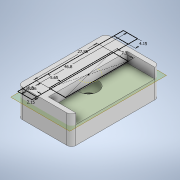
# Autodesk Inventor part: Capping_Parallelizer
Saved by Autodesk Inventor 2022 (Build 260153000, 153)
## iProperties
Created: 2024-04-15
Part Number: Capping_Parallelizer
Material: Generic
Document SubType Name: Modeling
Designer: Gotham City
Density: 1 g/cm^3
Appearance: Default
Author: Gotham City
Autodesk Inventor part; units mm, degrees
ref_plane "YZ Plane" through (0, 0, 0) normal (1, 0, 0) x (0, 1, 0)
ref_plane "XZ Plane" through (0, 0, 0) normal (0, 1, 0) x (-1, 0, 0)
sketch "Sketch1" plane through (0, 0, 0) normal (0, 1, 0) x (-1, 0, 0)
  line L0 (0, 0) -> (23.8, 0)
  line L1 (23.8, 0) -> (23.8, -39)
  line L2 (23.8, -39) -> (0, -39)
  line L3 (0, -39) -> (0, 0)
  circle A0 centre (11.9, -19.5) radius 9.9
  line L4 (23.8, 0) -> (0, -39) construction
  dimension "d0" = 19.8
  dimension "d1" = 11.9
  dimension "d2" = 39
  constraints: 10 end point, 2 parallel, 1 centre point, 1 coincident, 1 horizontal, 1 midpoint, 1 perpendicular
  measures "d0" diameter of A0
  measures "d1" distance from line of L1 A0.centre
  measures "d2" distance of L0.end L1.end
extrude "Extrusion1" add sketch "Sketch1" along normal blind 1.5
sketch "Sketch2" plane through (0, 0, 0) normal (0, -1, 0) x (1, 0, 0)
  line L0 (0, -39) -> (-23.8, -39) projected
  line L1 (0, 0) -> (0, -39) projected
  line L2 (-23.8, 0) -> (0, 0) projected
  line L3 (-23.8, -39) -> (-23.8, 0) projected
  circle A0 centre (-11.9, -19.5) radius 9.9 construction
  circle A1 centre (-11.9, -19.5) radius 4.25
  dimension "d5" = 8.5
  constraints: 1 centre point, 1 coincident
  measures "d5" diameter of A1
extrude "Extrusion2" add sketch "Sketch2" along normal blind 1
ref_plane "Work Plane1" through (0, 7, 0) normal (0, -1, 0) x (1, 0, 0)
sketch "Sketch4" plane through (0, 1.5, 0) normal (0, 1, 0) x (1, 0, 0)
  line L0 (0, 39) -> (-23.8, 39) projected
  line L1 (-23.8, 39) -> (-23.8, 0) projected
  line L2 (-23.8, 0) -> (0, 0) projected
  line L3 (0, 0) -> (0, 39) projected
  circle A0 centre (-11.9, 19.5) radius 4.25 projected
extrude "Extrusion3" add sketch "Sketch4" along normal up to surface (5.5 mm away)
sketch "Sketch5" plane through (-23.8, 7, -39) normal (0, 1, 0) x (1, 0, 0)
  line L0 (11.5916, -37) -> (27.5916, -37)
  line L1 (27.5916, -37) -> (27.5916, -2)
  line L2 (27.5916, -2) -> (11.5916, -2)
  line L3 (11.5916, -2) -> (11.5916, -37)
  line L4 (11.5916, -37) -> (27.5916, -2) construction
  line L5 (27.5916, -37) -> (11.5916, -2) construction
  line L6 (0, 0) -> (0, -39) projected
  line L7 (0, -39) -> (23.8, -39) projected
  line L8 (23.8, 0) -> (0, 0) projected
  line L9 (23.8, -39) -> (23.8, 0) projected
  dimension "d11" = 35
  dimension "d12" = 16
  constraints: 12 end point, 2 parallel, 1 horizontal, 1 perpendicular
  measures "d11" distance of L2.end L0.start
  measures "d12" distance of L0.start L0.end
extrude "Extrusion4" add sketch "Sketch5" along normal blind 4.5 contours L0 L9 L7 L6 L8 L2 L3
sketch "Sketch13" plane through (-23.8, 11.5, -39) normal (0, 1, 0) x (1, 0, 0)
  line L0 (8.9, -41.661) -> (2.6, -41.661)
  line L1 (2.6, -41.661) -> (2.6, 5.139)
  line L2 (2.6, 5.139) -> (8.9, 5.139)
  line L3 (8.9, 5.139) -> (8.9, -41.661)
  line L4 (8.25, -33.425) -> (8.25, -5.575) construction
  line L5 (15.55, -5.575) -> (8.25, -5.575)
  line L6 (8.25, -5.575) -> (8.25, -33.425)
  line L7 (8.25, -33.425) -> (15.55, -33.425)
  line L8 (15.55, -33.425) -> (15.55, -5.575)
  line L9 (15.55, -5.575) -> (8.25, -33.425) construction
  line L10 (8.25, -5.575) -> (15.55, -33.425) construction
  arc A0 (11.5916, -23.7388) -> (11.5916, -15.2612) centre (11.9, -19.5) ccw construction
  line L11 (2.6, 0.989) -> (8.9, 0.989)
  line L12 (8.9, -39.511) -> (2.6, -39.511)
  point P0 (11.9, -19.5)
  dimension "d62" = 5.65
  dimension "d63" = 46.8
  dimension "d64" = 6.3
  dimension "d65" = 8.236
  dimension "d66" = 27.85
  dimension "d67" = 7.3
  dimension "d74" = 4.15
  dimension "d75" = 2.15
  constraints: 26 end point, 4 perpendicular, 4 point on line, 3 horizontal, 3 midpoint, 3 parallel, 1 coincident
  measures "d62" distance between parallel lines of L1 L4
  measures "d63" distance of L0.end L1.end
  measures "d64" distance of L0.start L0.end
  measures "d65" distance from line of L0 L4.start
  measures "d66" distance between parallel lines of L5 L7
  measures "d67" distance of L5.start L4.end
  measures "d74" distance between parallel lines of L2 L11
  measures "d75" distance between parallel lines of L0 L12
thicken "Thicken1" operation add thickness 0.16 both sides no extend neighbours yes toward (0, -1, 0) faces at (-19.7796, 0, -20.6288)
fillet "Fillet1" radius 2 4 edges at (-23.8, 5.25, 0) (0, 5.25, 0) (0, 5.25, -39) (-23.8, 5.25, -39)
sketch "Sketch6" plane through (-23.8, 11.5, -39) normal (0, 1, 0) x (1, 0, 0)
  arc A0 (2, 0) -> (0, -2) centre (2, -2) ccw construction
  line L0 (0, -2) -> (0, -37) construction
  arc A1 (0, -37) -> (2, -39) centre (2, -37) ccw construction
  line L1 (2, -39) -> (21.8, -39) construction
  arc A2 (21.8, -39) -> (23.8, -37) centre (21.8, -37) ccw construction
  arc A3 (23.8, -2) -> (21.8, 0) centre (21.8, -2) ccw construction
  line L2 (21.8, 0) -> (2, 0) construction
  line L3 (11.5916, -37) -> (11.5916, -2) construction
  line L4 (11.5916, -2) -> (23.8, -2) construction
  line L5 (23.8, -37) -> (11.5916, -37) construction
  line L6 (8.9, -41.661) -> (2.6, -41.661) construction
  line L7 (-1.7, -43.661) -> (25.5, -43.661)
  line L8 (25.5, -43.661) -> (25.5, 7.139)
  line L9 (25.5, 7.139) -> (-1.7, 7.139)
  line L10 (-1.7, 7.139) -> (-1.7, -43.661)
  line L11 (2.6, 5.139) -> (8.9, 5.139) construction
  point P0 (23.8, -39)
  point P1 (11.9, -19.5)
  dimension "d69" = 2
  dimension "d70" = 2
  dimension "d71" = 1.7
  constraints: 8 end point, 2 parallel, 1 horizontal, 1 perpendicular
  measures "d69" distance between parallel lines of L7 L6
  measures "d70" distance between parallel lines of L9 L11
  measures "d71" distance between parallel lines of L0 L10
sketch "Sketch14" plane through (-23.8, 13, -39) normal (0, 1, 0) x (1, 0, 0)
  line L0 (8.9, -41.661) -> (2.6, -41.661) projected
  line L1 (2.6, 5.139) -> (8.9, 5.139) projected
  line L2 (25.5, 7.139) -> (-1.7, 7.139) projected
  line L3 (13.2, 7.139) -> (13.2, 0.989)
  line L4 (13.2, 0.989) -> (8.9, 0.989)
  line L5 (8.9, 0.989) -> (8.9, 5.139)
  line L6 (2.6, 5.139) -> (2.6, 0.989)
  line L7 (2.6, 0.989) -> (-1.7, 0.989)
  line L8 (-1.7, 7.139) -> (-1.7, -43.661) projected
  line L9 (-1.7, 0.989) -> (-1.7, 7.139)
  line L10 (-1.7, 7.139) -> (13.2, 7.139)
  line L11 (8.9, -39.511) -> (8.9, -41.661)
  line L12 (8.9, -39.511) -> (13.2, -39.511)
  line L13 (13.2, -39.511) -> (13.2, -43.661)
  line L14 (-1.7, -43.661) -> (25.5, -43.661) projected
  line L15 (13.2, -43.661) -> (-1.7, -43.661)
  line L16 (-1.7, -43.661) -> (-1.7, -39.511)
  line L17 (2.6, -39.511) -> (-1.7, -39.511)
  line L18 (2.6, -39.511) -> (2.6, -41.661)
  point P0 (23.8, -39)
  dimension "d76" = 4.3
  dimension "d77" = 4.3
  dimension "d78" = 4.3
  constraints: 28 end point, 9 perpendicular, 3 point on line, 2 vertical, 1 collinear, 1 horizontal
  measures "d76" distance of L3.end L4.end
  measures "d77" distance of L6.end L7.end
  measures "d78" distance of L11.start L12.end
sketch "Sketch15" plane through (-23.8, 13, -39) normal (0, 1, 0) x (1, 0, 0)
  line L0 (15.55, -5.575) -> (8.25, -5.575) projected
  line L1 (15.55, -33.425) -> (15.55, -5.575) projected
  line L2 (8.25, -33.425) -> (15.55, -33.425) projected
  line L3 (8.25, -5.575) -> (8.25, -33.425) projected
  point P0 (23.8, -39)
sketch "Sketch7" plane through (-23.8, 11.5, -39) normal (0, -1, 0) x (1, 0, 0)
  line L0 (0, 2) -> (0, 37) projected
  arc A0 (2, 39) -> (0, 37) centre (2, 37) ccw projected
  arc A1 (0, 2) -> (2, 0) centre (2, 2) ccw projected
  line L1 (21.8, 0) -> (2, 0) projected
  arc A2 (21.8, 0) -> (23.8, 2) centre (21.8, 2) ccw projected
  line L2 (23.8, 37) -> (23.8, 2) projected
  arc A3 (23.8, 37) -> (21.8, 39) centre (21.8, 37) ccw projected
  line L3 (2, 39) -> (21.8, 39) projected
  line L4 (-1.7, 43.661) -> (25.5, 43.661) projected
  line L5 (25.5, 43.661) -> (25.5, -7.139) projected
  line L6 (25.5, -7.139) -> (-1.7, -7.139) projected
  line L7 (-1.7, -7.139) -> (-1.7, 43.661) projected
sketch "Sketch8" plane through (0, -1, 0) normal (0, -1, 0) x (1, 0, 0)
  circle A0 centre (-11.9, -19.5) radius 4.25 construction
  circle A1 centre (-11.9, -19.5) radius 3.75
  point P0 (0, 0)
  dimension "d39" = 7.5
  dimension "d48" = 5
  dimension "d54" = 1
  constraints: 2 end point, 2 point on circle, 2 vertical alignment, 1 centre point, 1 midpoint, 1 vertical
sketch "Sketch12" plane through (-11.9, -3, -19.5) normal (0, 0, 1) x (1, 0, 0)
  line L0 (-3.2, 1) -> (-9.2, 1)
  line L1 (-9.2, 1) -> (-9.2, -0.75)
  line L2 (-9.2, -0.75) -> (-3.2, -0.75)
  line L3 (-3.2, -0.75) -> (-3.2, 1)
  line L4 (-3.75, 2) -> (3.75, 2) projected
  line L5 (0, 24.15) -> (0, -4.9) projected
  point P0 (11.9, 3)
  point P1 (-11.9, 0)
  point P2 (0, 2)
  point P3 (0, 1)
  dimension "d51" = 1.75
  dimension "d52" = 3.2
  dimension "d55" = 1
  dimension "d56" = 6
  constraints: 8 end point, 2 parallel, 1 horizontal, 1 midpoint, 1 vertical
  measures "d51" distance of L1.end L0.end
  measures "d52" distance from line of L3 point (0, 2)
  measures "d55" distance from line of L0 point (0, 2)
  measures "d56" distance of L0.start L0.end
sketch "Sketch16" plane through (-10.6, 12.7, 4.661) normal (0, 1, 0) x (1, 0, 0)
  line L0 (12.3, 0) -> (12.3, 50.8) projected
  line L1 (12.3, 50.8) -> (0, 50.8) projected
  line L2 (12.3, 0) -> (2.35, 0)
  line L3 (2.35, 0) -> (2.35, 50.8)
  line L4 (2.35, 50.8) -> (12.3, 50.8)
  line L5 (12.3, 50.8) -> (12.3, 0)
  point P0 (10.6, 4.661)
  point P1 (2.35, 38.086)
  constraints: 8 end point, 2 parallel, 2 point on line, 1 horizontal, 1 perpendicular
sketch "Sketch17" plane through (1.7, -1, 4.661) normal (1, 0, 0) x (0, 0, -1)
  line L0 (50.8, 12.3) -> (0, 12.3) projected
  line L1 (0, 12.3) -> (0, 0) projected
  line L2 (0, 0) -> (50.8, 0) projected
  line L3 (50.8, 0) -> (50.8, 12.3) projected
  point P0 (4.661, 1)
equation "\"d76\" = d77"
equation "\"d78\" = d77"
body "Solid1"
body "Solid2"
body "Solid3"
